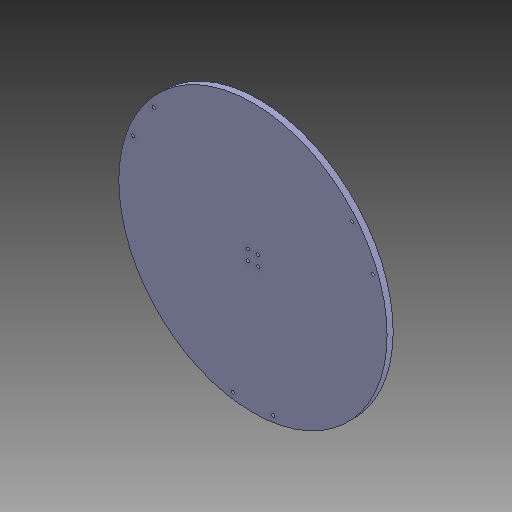
# Autodesk Inventor part: Диск опорный
Saved by Autodesk Inventor 2022 (Build 260153000, 153)
## iProperties
Created: 2025-01-11
Part Number: Диск опорный
Material: Типовые
Document SubType Name: Modeling
Designer: Ivan
Density: 1 g/cm^3
Appearance: Грифельно-синий
Mass: 330.445 g
Surface Area: 1157.47 cm^2
Volume: 330.445 cm^3
Author: Ivan
Title: Диск опорный
Autodesk Inventor part; units mm, degrees
ref_plane "YZ Plane" through (0, 0, 0) normal (1, 0, 0) x (0, 1, 0)
ref_plane "XZ Plane" through (0, 0, 0) normal (0, 1, 0) x (-1, 0, 0)
ref_plane "XY Plane" through (0, 0, 0) normal (0, 0, 1) x (1, 0, 0)
sketch "Эскиз1" plane through (0, 0, 0) normal (0, 0, 1) x (1, 0, 0)
  circle A0 centre (0, 0) radius 132.5
  dimension "d0" = 265
  constraints: 1 centre point, 1 coincident
  measures "d0" diameter of A0
extrude "Выдавливание1" add sketch "Эскиз1" along normal mid plane 6
sketch "Эскиз2" plane through (0, 0, -3) normal (0, 0, -1) x (-1, 0, 0)
  circle A0 centre (20, -124.909) radius 1.6 projected
  circle A1 centre (-20, -124.909) radius 1.6 projected
  point P0 (0, 0)
extrude "Выдавливание2" cut sketch "Эскиз2" against normal through all
pattern_circular "Круговой массив1" count 3 over 360 about axis through (0, 0, -10) along (0, 0, 1) of "Выдавливание2"
sketch "Эскиз3" plane through (0, 0, 3) normal (0, 0, 1) x (1, 0, 0)
  line L0 (-5, -5) -> (5, -5) construction
  line L1 (5, -5) -> (5, 5) construction
  line L2 (5, 5) -> (-5, 5) construction
  line L3 (-5, 5) -> (-5, -5) construction
  line L4 (-5, -5) -> (5, 5) construction
  line L5 (5, -5) -> (-5, 5) construction
  point P0 (0, 0)
  dimension "d8" = 10
  constraints: 12 end point, 4 coincident, 2 midpoint, 2 parallel, 2 perpendicular, 1 horizontal
  measures "d8" distance of L1.end L2.end
hole "Отверстие1" at (-5, 5, 3) at (5, 5, 3) at (-5, -5, 3) at (5, -5, 3) direction (0, 0, -1) diameter 3.2 end through all clearance for "болты с шестигранной головкой / гайка ГОСТ 12876-67" size "M3" standard "ГОСТ"
